lockingCircle (Autodesk Fusion 360 design; units mm, degrees)
Autodesk Fusion 360 part; units mm, degrees
sketch "Sketch1" plane through (0, 0, 0) normal (0, 0, 1) x (1, 0, 0)
  circle A0 centre (0, 0) radius 20
  circle A1 centre (0, 0) radius 15
  dimension "d1" = 40
  dimension "d2" = 30
  constraint coincident A0.centre A1.centre
  measures "d1" diameter of A0
  measures "d2" diameter of A1
extrude "Extrude1" add sketch "Sketch1" along normal blind 2.5
chamfer "Chamfer1" distance 1 angle 45 1 edges at (-18.6465, -7.2323, 0)
chamfer "Chamfer2" distance 1 angle 45 1 edges at (-13.9849, 5.4242, 0)
